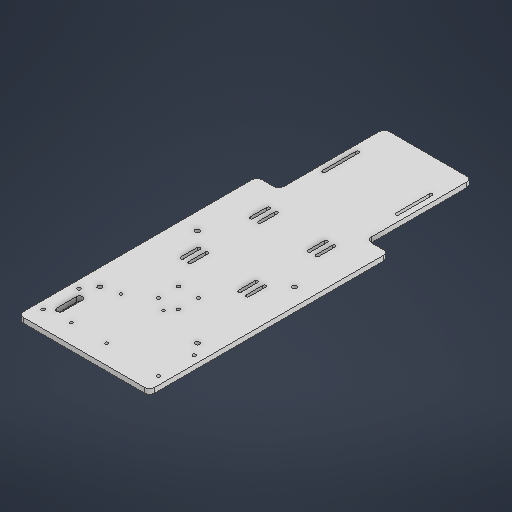
# Autodesk Inventor part: chassis
Saved by Autodesk Inventor 2026.1 (Build 301233000, 233)
## iProperties
Created: 2022-09-15
Part Number: chassis
Material: Générique
Document SubType Name: Modeling
Designer: ropertth
Density: 1 g/cm^3
Appearance: Par défaut
Mass: 199.944 g
Surface Area: 883.822 cm^2
Volume: 199.944 cm^3
Author: ropertth
## iProperties of the stored document chassis_3DPrint.ipt
Created: 2022-11-21
Part Number: chassis_3DPrint
Material: Generic
Document SubType Name: Modeling
Designer: Thomas
Density: 1 g/cm^3
Appearance: Default
Author: Thomas
Autodesk Inventor part; units mm, degrees
ref_plane "YZ Plane" through (0, 0, 0) normal (1, 0, 0) x (0, 1, 0)
ref_plane "XZ Plane" through (0, 0, 0) normal (0, 1, 0) x (-1, 0, 0)
ref_plane "XY Plane" through (0, 0, 0) normal (0, 0, 1) x (1, 0, 0)
sketch "Esquisse1" plane through (0, 0, 0) normal (0, 1, 0) x (-1, 0, 0)
  line L0 (66, 120) -> (-66, 120)
  line L1 (-66, 120) -> (-66, -120)
  line L2 (66, -120) -> (66, 120)
  line L3 (66, 120) -> (-66, -120) construction
  line L4 (-66, 120) -> (66, -120) construction
  line L5 (-44, -120) -> (-44, -226)
  line L6 (-44, -226) -> (44, -226)
  line L7 (44, -226) -> (44, -120)
  line L8 (-66, -120) -> (-44, -120)
  line L9 (44, -120) -> (66, -120)
  point P0 (0, 0)
  dimension "d0" = 240
  dimension "d1" = 132
  dimension "d2" = 88
  dimension "d3" = 44
  dimension "d5" = 346
  constraints: 20 end point, 4 parallel, 2 midpoint, 1 horizontal, 1 perpendicular
  measures "d0" distance of L2.start L0.start
  measures "d1" distance of L1.end L2.start
  measures "d2" distance of L5.end L6.end
  measures "d3" distance from line of point (0, 0) L7
  measures "d5" distance between parallel lines of L6 L0
extrude "Extrusion1" add sketch "Esquisse1" along normal blind 5
fillet "Congé1" radius 5 8 edges at (-66, 2.5, 120) (66, 2.5, 120) (66, 2.5, -120) (44, 2.5, -226) (44, 2.5, -120) (-44, 2.5, -226) (-44, 2.5, -120) (-66, 2.5, -120)
sketch "Esquisse3" plane through (0, 5, 0) normal (0, 1, 0) x (1, 0, 0)
  line L0 (-61, -120) -> (61, -120) projected
  line L1 (-66, 115) -> (-66, -115) projected
  point P0 (0, 0)
  point P1 (-58, -103)
  dimension "d31" = 17
  dimension "d32" = 8
  measures "d31" distance from line of L0 point (-58, -103)
  measures "d32" distance from line of L1 point (-58, -103)
hole "Perçage2" at (-58, 5, 103) direction (0, -1, 0) diameter 3.5 end through all
pattern_linear "Réseau rectangulaire2" count 2 spacing 36 along (0, 0, -1) count 2 spacing 116 along (1, 0, 0) of "Perçage2"
sketch "Esquisse4" plane through (0, 5, 0) normal (0, 1, 0) x (1, 0, 0)
  line L0 (-49.4, -75) -> (-49.4, -95) construction
  line L1 (-52.4, -75) -> (-52.4, -95)
  line L2 (-46.4, -95) -> (-46.4, -75)
  arc A0 (-46.4, -75) -> (-52.4, -75) centre (-49.4, -75) ccw
  arc A1 (-52.4, -95) -> (-46.4, -95) centre (-49.4, -95) ccw
  line L3 (66, -115) -> (66, 115) projected
  line L4 (-61, -120) -> (61, -120) projected
  line L5 (-66, 115) -> (-66, -115) projected
  point P0 (0, 0)
  point P1 (-49.4, -85)
  dimension "d39" = 3
  dimension "d41" = 35
  dimension "d42" = 20
  dimension "d45" = 16.6
  constraints: 8 end point, 4 point on circle, 4 tangent, 2 centre point, 1 midpoint, 1 parallel, 1 vertical
  measures "d39" radius of A1
  measures "d41" distance from line of L4 point (-49.4, -85)
  measures "d42" distance of L0.start L0.end
  measures "d45" distance between parallel lines of L5 L0
extrude "Extrusion2" cut sketch "Esquisse4" against normal through all
sketch "Esquisse5" plane through (0, 0, 0) normal (0, -1, 0) x (1, 0, 0)
  line L0 (-61, 120) -> (61, 120) projected
  line L1 (-66, -115) -> (-66, 115) projected
  point P0 (0, 0)
  point P1 (3.4, 100.5)
  dimension "d53" = 19.5
  dimension "d54" = 69.4
  measures "d53" distance from line of L0 point (3.4, 100.5)
  measures "d54" distance from line of L1 point (3.4, 100.5)
hole "Perçage3" at (3.4, 0, 100.5) direction (0, 1, 0) diameter 3 end through all
pattern_linear "Réseau rectangulaire3" count 2 spacing 57 along (0, 0, -1) of "Perçage3"
sketch "Esquisse6" plane through (0, 0, 0) normal (0, -1, 0) x (1, 0, 0)
  line L0 (-61, 120) -> (61, 120) projected
  line L1 (-66, -115) -> (-66, 115) projected
  point P0 (0, 0)
  point P1 (-32.3, 100.5)
  dimension "d65" = 19.5
  dimension "d66" = 33.7
  measures "d65" distance from line of L0 point (-32.3, 100.5)
  measures "d66" distance from line of L1 point (-32.3, 100.5)
hole "Perçage4" at (-32.3, 0, 100.5) direction (0, 1, 0) diameter 3 end through all
pattern_linear "Réseau rectangulaire4" count 2 spacing 50 along (0, 0, -1) of "Perçage4"
sketch "Esquisse7" plane through (0, 0, 0) normal (0, -1, 0) x (1, 0, 0)
  line L0 (-37, -192) -> (-37, -158) construction
  line L1 (-38.5, -192) -> (-38.5, -158)
  line L2 (-35.5, -158) -> (-35.5, -192)
  arc A0 (-38.5, -192) -> (-35.5, -192) centre (-37, -192) ccw
  arc A1 (-35.5, -158) -> (-38.5, -158) centre (-37, -158) ccw
  line L3 (39, -226) -> (-39, -226) projected
  line L4 (-44, -221) -> (-44, -125) projected
  point P0 (0, 0)
  point P1 (-37, -175)
  dimension "d70" = 1.5
  dimension "d71" = 34
  dimension "d72" = 34
  dimension "d73" = 7
  constraints: 8 end point, 4 point on circle, 4 tangent, 2 centre point, 1 midpoint, 1 parallel, 1 vertical
  measures "d70" radius of A1
  measures "d71" distance from line of L3 L0.start
  measures "d72" distance of L0.start L0.end
  measures "d73" distance between parallel lines of L0 L4
extrude "Extrusion3" cut sketch "Esquisse7" against normal through all
mirror "Symétrie1" about plane through (0, 0, 0) normal (1, 0, 0) of "Extrusion3"
sketch "Sketch8" plane through (0, 5, 0) normal (0, 1, 0) x (1, 0, 0)
  line L0 (-61, -120) -> (61, -120) construction
  line L1 (0, -120) -> (0, 226) construction
  line L2 (39, 226) -> (-39, 226) construction
  point P0 (0, 0)
  point P1 (49, -55)
  point P2 (49, 43)
  point P3 (-49, -55)
  point P4 (-49, 43)
  dimension "d86" = 98
  dimension "d89" = 98
  dimension "d92" = 49
  dimension "d93" = 65
  constraints: 2 end point, 2 midpoint, 1 horizontal, 1 vertical, 3 other
  measures "d86" distance of point (49, -55) point (49, 43)
  measures "d89" distance of point (49, -55) point (-49, -55)
  measures "d92" distance from line of L1 point (49, -55)
  measures "d93" distance from line of L0 point (49, -55)
hole "Hole5" at (49, 5, 55) at (49, 5, -43) at (-49, 5, 55) at (-49, 5, -43) direction (0, -1, 0) diameter 4.5 end through all clearance for "Countersunk Flat Head Screw DIN EN ISO 2009" size "M4" standard "DIN"
sketch "Sketch9" plane through (0, 5, 0) normal (0, 1, 0) x (1, 0, 0)
  line L0 (25, 11.5) -> (25, 28.5) construction
  line L1 (26.5, 11.5) -> (26.5, 28.5)
  line L2 (23.5, 28.5) -> (23.5, 11.5)
  arc A0 (23.5, 11.5) -> (26.5, 11.5) centre (25, 11.5) ccw
  arc A1 (26.5, 28.5) -> (23.5, 28.5) centre (25, 28.5) ccw
  line L3 (0, 0) -> (47.7976, 0) construction
  line L4 (33, 11.5) -> (33, 28.5) construction
  line L5 (34.5, 11.5) -> (34.5, 28.5)
  line L6 (31.5, 28.5) -> (31.5, 11.5)
  arc A2 (31.5, 11.5) -> (34.5, 11.5) centre (33, 11.5) ccw
  arc A3 (34.5, 28.5) -> (31.5, 28.5) centre (33, 28.5) ccw
  line L7 (0, 0) -> (0, 64.8348) construction
  line L8 (-25, 11.5) -> (-25, 28.5) construction
  line L9 (-33, 11.5) -> (-33, 28.5) construction
  line L10 (-31.5, 11.5) -> (-31.5, 28.5)
  line L11 (-34.5, 28.5) -> (-34.5, 11.5)
  line L12 (-26.5, 28.5) -> (-26.5, 11.5)
  line L13 (-23.5, 11.5) -> (-23.5, 28.5)
  arc A4 (-34.5, 11.5) -> (-31.5, 11.5) centre (-33, 11.5) ccw
  arc A5 (-26.5, 11.5) -> (-23.5, 11.5) centre (-25, 11.5) ccw
  arc A6 (-31.5, 28.5) -> (-34.5, 28.5) centre (-33, 28.5) ccw
  arc A7 (-23.5, 28.5) -> (-26.5, 28.5) centre (-25, 28.5) ccw
  line L14 (33, 81.5) -> (33, 98.5) construction
  line L15 (25, 81.5) -> (25, 98.5) construction
  line L16 (26.5, 81.5) -> (26.5, 98.5)
  line L17 (23.5, 98.5) -> (23.5, 81.5)
  line L18 (31.5, 98.5) -> (31.5, 81.5)
  line L19 (34.5, 81.5) -> (34.5, 98.5)
  arc A8 (23.5, 81.5) -> (26.5, 81.5) centre (25, 81.5) ccw
  arc A9 (31.5, 81.5) -> (34.5, 81.5) centre (33, 81.5) ccw
  arc A10 (26.5, 98.5) -> (23.5, 98.5) centre (25, 98.5) ccw
  arc A11 (34.5, 98.5) -> (31.5, 98.5) centre (33, 98.5) ccw
  line L20 (-25, 81.5) -> (-25, 98.5) construction
  line L21 (-33, 81.5) -> (-33, 98.5) construction
  line L22 (-31.5, 81.5) -> (-31.5, 98.5)
  line L23 (-34.5, 98.5) -> (-34.5, 81.5)
  line L24 (-26.5, 98.5) -> (-26.5, 81.5)
  line L25 (-23.5, 81.5) -> (-23.5, 98.5)
  arc A12 (-34.5, 81.5) -> (-31.5, 81.5) centre (-33, 81.5) ccw
  arc A13 (-26.5, 81.5) -> (-23.5, 81.5) centre (-25, 81.5) ccw
  arc A14 (-31.5, 98.5) -> (-34.5, 98.5) centre (-33, 98.5) ccw
  arc A15 (-23.5, 98.5) -> (-26.5, 98.5) centre (-25, 98.5) ccw
  point P0 (25, 20)
  point P1 (25, 10)
  point P2 (25, 30)
  point P3 (33, 10)
  point P4 (33, 30)
  point P5 (33, 20)
  point P6 (-33, 20)
  point P7 (-25, 20)
  point P8 (-33, 10)
  point P9 (-25, 10)
  point P10 (-33, 30)
  point P11 (-25, 30)
  point P12 (25, 90)
  point P13 (33, 90)
  point P14 (25, 80)
  point P15 (33, 80)
  point P16 (25, 100)
  point P17 (33, 100)
  point P18 (-33, 90)
  point P19 (-25, 90)
  point P20 (-33, 80)
  point P21 (-25, 80)
  point P22 (-33, 100)
  point P23 (-25, 100)
  dimension "d94" = 3
  dimension "d95" = 20
  dimension "d96" = 25
  dimension "d99" = 8
  dimension "d115" = 58
  dimension "d118" = 70
  dimension "d123" = 20
  constraints: 68 end point, 34 point on circle, 16 centre point, 4 tangent, 3 horizontal, 3 vertical, 1 midpoint, 1 parallel, 98 other
  measures "d94" distance between parallel lines of L1 L2
  measures "d95" distance of point (25, 10) point (25, 30)
  measures "d96" distance from line of L0 L3.start
  measures "d99" distance of L1.start L5.start
  measures "d115" distance of L1.end L10.end
  measures "d118" distance of L1.end L16.end
  measures "d123" distance from line of L3 point (25, 20)
extrude "Extrusion4" cut sketch "Sketch9" against normal through all
sketch "Sketch11" plane through (0, 5, 0) normal (0, 1, 0) x (1, 0, 0)
  line L0 (0, 0) -> (22.9604, 0) construction
  line L1 (22.9604, 0) -> (0, 0) construction
  line L2 (0, 13.4889) -> (0, 0) construction
  point P0 (-10, -35)
  point P1 (10, -35)
  point P2 (-10, -15)
  point P3 (10, -15)
  dimension "d131" = 10
  dimension "d132" = 35
  dimension "d135" = 20
  dimension "d138" = 20
  constraints: 6 end point, 2 horizontal, 1 collinear, 1 perpendicular, 1 vertical, 3 other
  measures "d131" horizontal distance of L0.start point (-10, -35)
  measures "d132" vertical distance of L0.start point (-10, -35)
  measures "d135" distance of point (-10, -35) point (10, -35)
  measures "d138" distance of point (-10, -35) point (-10, -15)
hole "Hole6" at (-10, 5, 35) at (10, 5, 35) at (-10, 5, 15) at (10, 5, 15) direction (0, -1, 0) diameter 3.4 end through all clearance for "Countersunk Flat Head Screw DIN EN ISO 2009" size "M3" standard "DIN"
equation "\"d86\" = pcb_fixation_ecart"
equation "\"d89\" = pcb_fixation_ecart"
equation "\"d92\" = 0.5 * d89"
equation "\"d115\" = 2 * d96 + d99"
equation "\"d135\" = 2 * d131"
equation "\"pcb_fixation_ecart\" = 98"
